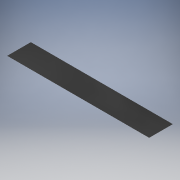
# Autodesk Inventor part: Panel
Saved by Autodesk Inventor 2017.2 (Build 212233000, 233)
## iProperties
Created: 2017-03-31
Part Number: Panel
Material: Silicon Nitride
Document SubType Name: Modeling
Designer: haden
Density: 3.18 g/cm^3
Appearance: Chrome - Polished Black
Author: haden
Autodesk Inventor part; units mm, degrees
ref_plane "YZ Plane" through (0, 0, 0) normal (1, 0, 0) x (0, 1, 0)
ref_plane "XZ Plane" through (0, 0, 0) normal (0, 1, 0) x (-1, 0, 0)
ref_plane "XY Plane" through (0, 0, 0) normal (0, 0, 1) x (1, 0, 0)
sketch "Sketch1" plane through (0, 0, 0) normal (0, 1, 0) x (-1, 0, 0)
  line L0 (0, 0) -> (-300000, 0)
  line L1 (-300000, 0) -> (-300000, -50000)
  line L2 (-300000, -50000) -> (0, -50000)
  line L3 (0, -50000) -> (0, 0)
  dimension "d0" = 300000
  dimension "d1" = 50000
  constraints: 8 end point, 2 parallel, 1 horizontal, 1 perpendicular
  measures "d0" distance of L2.end L1.end
  measures "d1" distance of L1.end L0.end
extrude "Extrusion1" add sketch "Sketch1" along normal blind 100
body "Solid1"
